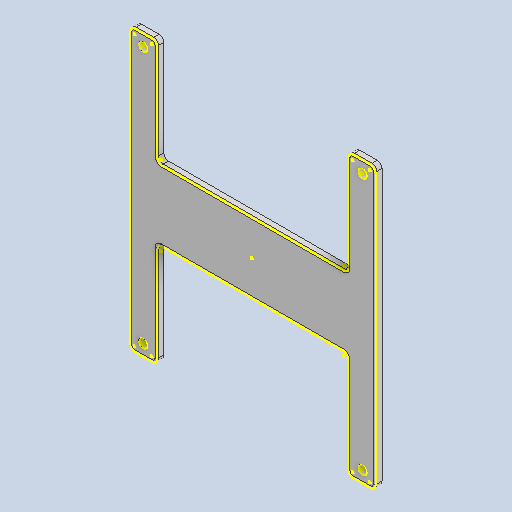
# Autodesk Inventor part: BatteryHolderTop
Saved by Autodesk Inventor 2022 (Build 260153000, 153)
## iProperties
Created: 2021-02-16
Part Number: BatteryHolderTop
Material: Generic
Document SubType Name: Modeling
Designer: Viktor
Density: 1 g/cm^3
Appearance: Default
Author: Viktor
Autodesk Inventor part; units mm, degrees
ref_plane "YZ Plane" through (0, 0, 0) normal (1, 0, 0) x (0, 1, 0)
ref_plane "XZ Plane" through (0, 0, 0) normal (0, 1, 0) x (-1, 0, 0)
ref_plane "XY Plane" through (0, 0, 0) normal (0, 0, 1) x (1, 0, 0)
sketch "Sketch1" plane through (0, 0, 0) normal (0, 0, 1) x (1, 0, 0)
  line L0 (-52.5, -60) -> (52.5, -60)
  line L1 (52.5, -60) -> (52.5, 60)
  line L2 (52.5, 60) -> (-52.5, 60)
  line L3 (-52.5, 60) -> (-52.5, -60)
  line L4 (-52.5, -60) -> (52.5, 60) construction
  line L5 (52.5, -60) -> (-52.5, 60) construction
  point P0 (0, 0)
  dimension "d0" = 105
  dimension "d1" = 120
  constraints: 12 end point, 2 midpoint, 2 parallel, 1 horizontal, 1 perpendicular
  measures "d0" distance between parallel lines of L1 L3
  measures "d1" distance between parallel lines of L0 L2
extrude "Extrusion1" add sketch "Sketch1" along normal blind 3
sketch "Sketch2" plane through (0, 0, 3) normal (0, 0, 1) x (1, 0, 0)
  circle A0 centre (-47, 55) radius 1.75
  line L0 (-73.5, 0) -> (73.5, 0) construction
  line L1 (0, 84) -> (0, -84) construction
  circle A1 centre (47, 55) radius 1.75
  circle A2 centre (-47, -55) radius 1.75
  circle A3 centre (47, -55) radius 1.75
  point P0 (0, 0)
  dimension "d4" = 3.5
  dimension "d5" = 94
  dimension "d6" = 110
  constraints: 4 centre point, 3 symmetric about line, 3 other
  measures "d4" diameter of A0
  measures "d5" distance of A1.centre A0.centre
  measures "d6" distance of A2.centre A0.centre
extrude "Extrusion2" cut sketch "Sketch2" against normal blind 3
sketch "Sketch3" plane through (0, 0, 3) normal (0, 0, 1) x (1, 0, 0)
  line L0 (52.5, 60) -> (-52.5, 60) construction
  line L1 (52.5, 60) -> (-52.5, 60) construction
  line L2 (-41, 60) -> (41, 60)
  line L3 (41, 60) -> (41, 15)
  line L4 (41, 15) -> (-41, 15)
  line L5 (-41, 15) -> (-41, 60)
  line L6 (-52.5, 60) -> (-52.5, -60) construction
  line L7 (52.5, -60) -> (52.5, 60) construction
  line L8 (-73.5, 0) -> (73.5, 0) projected
  line L9 (52.5, -60) -> (-52.5, -60) construction
  line L10 (52.5, -60) -> (-52.5, -60) construction
  line L11 (-41, -60) -> (41, -60)
  line L12 (41, -60) -> (41, -15)
  line L13 (41, -15) -> (-41, -15)
  line L14 (-41, -15) -> (-41, -60)
  point P0 (0, 0)
  dimension "d9" = 15
  dimension "d10" = 82
  dimension "d11" = 11.5
  dimension "d12" = 105
  constraints: 20 end point, 4 symmetric about line, 2 parallel, 2 point on line, 1 horizontal, 1 perpendicular
  measures "d9" distance from line of point (0, 0) L4
  measures "d10" distance between parallel lines of L3 L5
  measures "d11" distance between parallel lines of L5 L6
  measures "d12" distance between parallel lines of L7 L6
extrude "Extrusion3" cut sketch "Sketch3" against normal blind 3
fillet "Fillet1" radius 2 4 edges at (-41, 15, 1.5) (41, 15, 1.5) (41, -15, 1.5) (-41, -15, 1.5)
fillet "Fillet2" radius 2 8 edges at (41, 60, 1.5) (52.5, 60, 1.5) (-41, 60, 1.5) (-52.5, 60, 1.5) (-52.5, -60, 1.5) (-41, -60, 1.5) (41, -60, 1.5) (52.5, -60, 1.5)
chamfer "Chamfer1" distance 0.75 angle 45 24 edges at (52.5, 0, 3) (51.9142, 59.4142, 3) (46.75, 60, 3) (41.5858, 59.4142, 3) (41, 37.5, 3) (40.4142, 15.5858, 3) (0, 15, 3) (-40.4142, 15.5858, 3) (-41, 37.5, 3) (-41.5858, 59.4142, 3) (-46.75, 60, 3) (-51.9142, 59.4142, 3) (-52.5, 0, 3) (-51.9142, -59.4142, 3) (-46.75, -60, 3) (-41.5858, -59.4142, 3) (-41, -37.5, 3) (-40.4142, -15.5858, 3) (0, -15, 3) (40.4142, -15.5858, 3) (41, -37.5, 3) (41.5858, -59.4142, 3) (46.75, -60, 3) (51.9142, -59.4142, 3)
sketch "Sketch4" plane through (0, 0, 3) normal (0, 0, 1) x (1, 0, 0)
  line L0 (-41, 17) -> (-41, 58) projected
  arc A0 (-41, 17) -> (-39, 15) centre (-39, 17) ccw projected
  line L1 (39, 15) -> (-39, 15) projected
  arc A1 (39, 15) -> (41, 17) centre (39, 17) ccw projected
  line L2 (41, 58) -> (41, 17) projected
  arc A2 (43, 60) -> (41, 58) centre (43, 58) ccw projected
  line L3 (50.5, 60) -> (43, 60) projected
  arc A3 (52.5, 58) -> (50.5, 60) centre (50.5, 58) ccw projected
  line L4 (52.5, -58) -> (52.5, 58) projected
  arc A4 (50.5, -60) -> (52.5, -58) centre (50.5, -58) ccw projected
  line L5 (43, -60) -> (50.5, -60) projected
  arc A5 (41, -58) -> (43, -60) centre (43, -58) ccw projected
  line L6 (41, -17) -> (41, -58) projected
  arc A6 (41, -17) -> (39, -15) centre (39, -17) ccw projected
  line L7 (-39, -15) -> (39, -15) projected
  arc A7 (-39, -15) -> (-41, -17) centre (-39, -17) ccw projected
  line L8 (-41, -58) -> (-41, -17) projected
  arc A8 (-43, -60) -> (-41, -58) centre (-43, -58) ccw projected
  line L9 (-50.5, -60) -> (-43, -60) projected
  arc A9 (-52.5, -58) -> (-50.5, -60) centre (-50.5, -58) ccw projected
  line L10 (-52.5, 58) -> (-52.5, -58) projected
  arc A10 (-50.5, 60) -> (-52.5, 58) centre (-50.5, 58) ccw projected
  line L11 (-43, 60) -> (-50.5, 60) projected
  arc A11 (-41, 58) -> (-43, 60) centre (-43, 58) ccw projected
  circle A12 centre (-47, 55) radius 1.75 projected
  circle A13 centre (47, 55) radius 1.75 projected
  circle A14 centre (47, -55) radius 1.75 projected
  circle A15 centre (-47, -55) radius 1.75 projected
  point P0 (0, 0)
equation "\"d11\" = -0.5 * d10 + 0.5 * d12"
body "Solid1"
